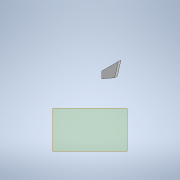
# Autodesk Inventor part: LegConnector
Saved by Autodesk Inventor 2022 (Build 260153000, 153)
## iProperties
Created: 2021-12-19
Part Number: LegConnector
Material: Generic
Document SubType Name: Modeling
Designer: dangl
Density: 1 g/cm^3
Appearance: Default
Author: dangl
Autodesk Inventor part; units mm, degrees
ref_plane "YZ Plane" through (0, 0, 0) normal (1, 0, 0) x (0, 1, 0)
ref_plane "XZ Plane" through (0, 0, 0) normal (0, 1, 0) x (-1, 0, 0)
ref_plane "XY Plane" through (0, 0, 0) normal (0, 0, 1) x (1, 0, 0)
sketch "Sketch1" plane through (0, 0, 0) normal (0, 0, 1) x (1, 0, 0)
  line L0 (3.7914, 27.5) -> (2.2914, 27.5) projected
  line L1 (2.2914, 27.5) -> (-3.9695, 0.5) projected
  line L2 (-3.9695, 0.5) -> (-0.9695, 0.5) projected
  line L3 (-0.9695, 0.5) -> (3.7914, 27.5) projected
  line L4 (-0.4912, 15.5) -> (-6.1042, 12.2594)
  line L5 (0.6682, 20.5) -> (-6.1042, 13.7277)
  line L6 (-0.4912, 15.5) -> (0.6682, 20.5)
  line L7 (-6.1042, 12.2594) -> (-6.1042, 13.7277)
  point P0 (0, 0)
  dimension "d0" = 30
  dimension "d1" = 45
  dimension "d2" = 15
  dimension "d3" = 20
  constraints: 8 end point, 2 point on line, 1 collinear, 1 vertical
  measures "d0" angle of L2 L4
  measures "d1" angle of L5 L2
  measures "d2" distance from line of L2 L4.start
  measures "d3" distance from line of L2 L5.start
extrude "Extrusion1" add sketch "Sketch1" along normal mid plane 0.8 contours L1 L4 L7 L5
ref_plane "Work Plane1" through (-6.8792, -1.2, 1.7678) normal (0, -1, 0) x (-0.7071068, 0, -0.7071068)
sketch "Sketch2" plane through (-6.8792, -1.2, 1.7678) normal (0, -1, 0) x (-0.7071068, 0, -0.7071068)
  line L0 (-5, 7.5) -> (-5, -7.5) projected
  line L1 (-5, -7.5) -> (5, -7.5) projected
  line L2 (5, -7.5) -> (5, 7.5) projected
  line L3 (5, 7.5) -> (-5, 7.5) projected
  line L4 (5, 7.5) -> (-5, -7.5)
  line L5 (5, -7.5) -> (0, 0)
  line L6 (0.9848, 2.0809) -> (-3.804, 6.8697) projected
  line L7 (-0.125, 3.1907) -> (-0.6907, 2.625)
  line L8 (0.4191, 1.5152) -> (-3.5499, 5.4842) projected
  line L9 (0, 0) -> (-5, 7.5)
  line L10 (0.9848, 2.0809) -> (-0.125, 3.1907)
  line L11 (0.4191, 1.5152) -> (-0.6907, 2.625)
  line L12 (0.9848, 2.0809) -> (0.4191, 1.5152)
  point P0 (-3.6144, 6.1144)
  dimension "d6" = 0.125
  constraints: 14 end point, 3 point on line, 2 perpendicular, 1 midpoint, 1 parallel
  measures "d6" horizontal distance of L7.start L5.end
extrude "Extrusion2" cut sketch "Sketch2" against normal through all contours L12 L8 L7 L6
body "Solid1"
